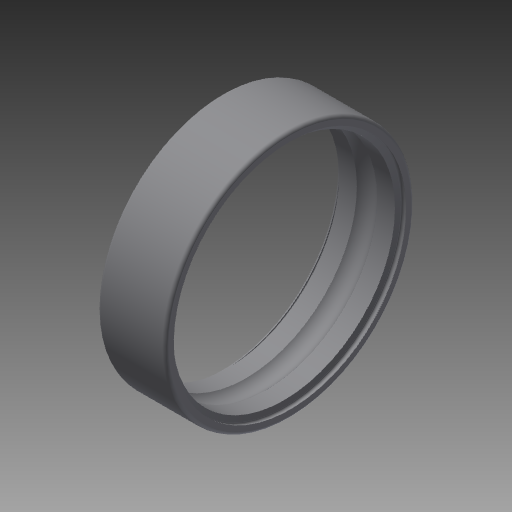
# Autodesk Inventor part: W 627/7-2ZS_PART2
Saved by Autodesk Inventor 2019.1 (Build 231200000, 200)
## iProperties
Category: PARTsolutions
Company: SKF
Created: 2018-12-01
Part Number: W 627/7-2ZS_PART2
Material: Allgemein
Catalog Web Link: www.cadenas.de
Description: -Deep groove ball bearings
Vendor: SKF
Document SubType Name: Modeling
Designer: psadmin
Manufacturer: SKF
Mass: 0.0501247 g
Surface Area: 2.40209 cm^2
Volume: 0.0501247 cm^3
Density: 1 g/cm^3
Appearance: PSOLRGB-175-175-175
PSOL_IDENT_0: {$CADENAS_DATA\23d-libs\skf\bearings_units_and_housings\ball_bearings\deep_groove_ball_bearings\bb1_
PSOL_IDENT_1: 001_101.prj},201 {VTYP=3D},{NB=W 627/7-2ZS_PART2},{LINA=W 627/7-2ZS_PART2},{NN=BB1_001_101_PART2},{N
PSOL_IDENT_2: OPRJ=TRUE},{DATE=29.11.2018 10:40:58},{GEOMDATE=08.08.2018 12:16:40},{VERSION=},{LINEID=19830},{WBVA
PSOL_IDENT_3: R=},{WBNUMERIC=}  {NB=W 627/7-2ZS_PART2},{LINA=W 627/7-2ZS_PART2},{KT=DUMMY},{PRODUCTID=},{DESIGNATI
PSOL_IDENT_4: ON=W 627/7-2ZS},{DD=7.00},{D=11.000},{B=3.000},{C=0.000},{DD1=8.04},{DD2=0.0},{D1=0.00},{D2=10.26},{
PSOL_IDENT_5: D3=0.00},{D4=0.000},{HH=MIN},{BB=0.000},{FF=0.00},{R0MAX=MIN},{R0=MIN},{R12=0.15},{PITCH=9.00},{DW=1
PSOL_IDENT_6: .200},{DDAMIN=7.900},{DDAMAX=7.900},{DDBMIN=MIN},{DDBMAX=MIN},{DBMIN=MIN},{DAMAX=10.300},{BBAMIN=MIN
PSOL_IDENT_7: },{CAMAX=MIN},{RAMAX=0.150},{LOAD1=0.260},{LOAD2=0.104},{LOAD3=0.004},{SPEED1=110000},{SPEED2=56000}
PSOL_IDENT_8: ,{KR=0.015},{F0=8.100},{Z=9},{II=1},{MASS=0.001},{BEARING=W 627/7-2ZS},{RING=},{HELP=0.598},{HELP2=0
PSOL_IDENT_9: .370},{DD1ALG=4.020},{YALG=4.020},{PITCH1=9.000},{DW1=1.200},{YALG1=4.902},{HALG1=0.598},{SH=4.020},
PSOL_IDENT_10: {CU=0.360},{DESIGN=dgbbw2z},{HALG=0.52},{B1=0},{ALGO=1.000}
NT: Deep groove ball bearings
NB: W 627/7-2ZS_PART2
NBSYN: $DESIGNATION._PART2
LINA: W 627/7-2ZS_PART2
SUPPLIER: SKF
ARTICLENO: W 627/7-2ZS_PART2
BOMINFO: W 627/7-2ZS_PART2
CREATOR: CADENAS GmbH
Title: W 627/7-2ZS_PART2
Author: Cadenas PARTsolutions
Comments: Deep groove ball bearings
Autodesk Inventor part; units mm, degrees
ref_plane "YZ Plane" through (0, 0, 0) normal (1, 0, 0) x (0, 1, 0)
ref_plane "XZ Plane" through (0, 0, 0) normal (0, 1, 0) x (-1, 0, 0)
ref_plane "XY Plane" through (0, 0, 0) normal (0, 0, 1) x (1, 0, 0)
sketch "Sketch_17" plane through (0, 0, 0) normal (0, 0, 1) x (1, 0, 0)
  line L0 (50, 0) -> (-50, 0)
  line L1 (0, 5.35) -> (0, 5.13)
  line L2 (0, 5.13) -> (0.045, 5.13)
  arc A0 (0.225, 5.13) -> (0.045, 5.13) centre (0.135, 5.13) ccw
  line L3 (0.225, 5.13) -> (0.2652, 4.902)
  line L4 (0.2652, 4.902) -> (1.0546, 4.902)
  arc A1 (1.9454, 4.902) -> (1.0546, 4.902) centre (1.5, 4.5) ccw
  line L5 (1.9454, 4.902) -> (2.7348, 4.902)
  line L6 (2.7348, 4.902) -> (2.775, 5.13)
  arc A2 (2.955, 5.13) -> (2.775, 5.13) centre (2.865, 5.13) ccw
  line L7 (2.955, 5.13) -> (3, 5.13)
  line L8 (3, 5.13) -> (3, 5.35)
  arc A3 (3, 5.35) -> (2.85, 5.5) centre (2.85, 5.35) ccw
  line L9 (2.85, 5.5) -> (0.15, 5.5)
  arc A4 (0.15, 5.5) -> (0, 5.35) centre (0.15, 5.35) ccw
  constraints: 20 end point, 10 point on circle, 5 centre point
revolve "Revolution1" add sketch "Sketch_17" angle 360 about axis through (50, 0, 0) along (1, 0, 0)
body "Solid1"
